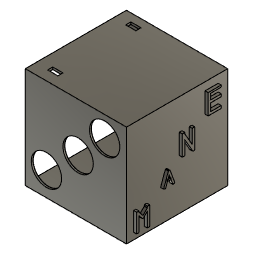
Trabalho #01 (Autodesk Fusion 360 design; units mm, degrees)
Autodesk Fusion 360 part; units mm, degrees
sketch "Sketch1" plane through (0, 0, 0) normal (0, 0, 1) x (1, 0, 0)
  line L0 (2.4742, 2.2756) -> (97.4742, 2.2756)
  line L1 (97.4742, 2.2756) -> (97.4742, 97.2756)
  line L2 (97.4742, 97.2756) -> (2.4742, 97.2756)
  line L3 (2.4742, 97.2756) -> (2.4742, 2.2756)
  line L4 (0, 0) -> (100, 0)
  line L5 (100, 0) -> (100, 100)
  line L6 (100, 100) -> (0, 100)
  line L7 (0, 100) -> (0, 0)
  dimension "d1" = 95
  dimension "d2" = 95
  dimension "d3" = 100
  dimension "d4" = 100
  constraint horizontal L0
  constraint vertical L1
  constraint horizontal L2
  constraint vertical L3
  constraint horizontal L4
  constraint vertical L5
  constraint horizontal L6
  constraint vertical L7
  constraint coincident L4.start L7.end
  measures "d1" distance of L0.start L0.end
  measures "d2" distance of L0.start L2.end
  measures "d3" distance of L4.start L4.end
  measures "d4" distance of L4.start L6.end
extrude "Extrude1" add sketch "Sketch1" along normal blind 113 contours L0 L1 L2 L3 makes body 1
sketch "Sketch2" plane through (0, 0, 0) normal (0, 0, 1) x (1, 0, 0)
  line L0 (0, 0) -> (100, 0)
  line L1 (100, 0) -> (100, 100)
  line L2 (100, 100) -> (0, 100)
  line L3 (0, 100) -> (0, 0)
  dimension "d7" = 100
  dimension "d8" = 100
  constraint horizontal L0
  constraint vertical L1
  constraint horizontal L2
  constraint vertical L3
  constraint coincident L0.start L3.end
  measures "d7" distance of L0.start L0.end
  measures "d8" distance of L0.start L2.end
extrude "Extrude2" cut sketch "Sketch2" along normal blind 113.5 bodies 1
sketch "Sketch3" plane through (0, 0, 0) normal (0, 1, 0) x (1, 0, 0)
  line L0 (0, 0) -> (100, 0)
  line L1 (100, 0) -> (100, -100)
  line L2 (100, -100) -> (0, -100)
  line L3 (0, -100) -> (0, 0)
  dimension "d11" = 100
  dimension "d12" = 100
  constraint horizontal L0
  constraint vertical L1
  constraint horizontal L2
  constraint vertical L3
  constraint coincident L0.start L3.end
  measures "d11" distance of L0.start L0.end
  measures "d12" distance of L0.start L2.end
extrude "Extrude3" add sketch "Sketch3" along normal blind 100 bodies 1
sketch "Sketch4" plane through (0, 0, 0) normal (0, 0, 1) x (1, 0, 0)
  line L0 (0, 0) -> (-96, 0)
  line L1 (-96, 0) -> (-96, -96)
  line L2 (-96, -96) -> (0, -96)
  line L3 (0, -96) -> (0, 0)
  dimension "d15" = 96
  dimension "d16" = 96
  constraint horizontal L0
  constraint vertical L1
  constraint horizontal L2
  constraint vertical L3
  constraint coincident L0.start L3.end
  measures "d15" distance of L0.start L0.end
  measures "d16" distance of L0.start L2.end
extrude "Extrude4" add sketch "Sketch4" along normal blind 96 separate body makes body 2
move_body "Move1" bodies 2 to x (1, 0, 0) y (0, 1, 0) z (0, 0, 1) at (51.5618, 26.4933, 12.8191)
move_body "Move2" bodies 2 to x (1, 0, 0) y (0, 1, 0) z (0, 0, 1) at (30.545, 71.415, -8.7648)
move_body "Move3" bodies 2 to x (1, 0, 0) y (0, 1, 0) z (0, 0, 1) at (-126.1069, -2.5329, 0.0199)
move_body "Move4" bodies 2 to x (1, 0, 0) y (0, 1, 0) z (0, 0, 1) at (14.4031, -1.4043, 59.8669)
move_body "Move5" bodies 2 to x (1, 0, 0) y (0, 1, 0) z (0, 0, 1) at (-24.3693, 162.9476, 0)
move_body "Move6" bodies 2 to x (1, 0, 0) y (0, 1, 0) z (0, 0, 1) at (110, 0, 0)
move_body "Move7" bodies 2 to x (1, 0, 0) y (0, 1, 0) z (0, 0, 1) at (0, -160, -65)
move_body "Move8" bodies 2 to x (1, 0, 0) y (0, 1, 0) z (0, 0, 1) at (0.0912, 0.7995, 1.9212)
move_body "Move9" bodies 2 to x (1, 0, 0) y (0, 1, 0) z (0, 0, 1) at (42.5, 0, 1)
sketch "Sketch5" plane through (0, 0, 0) normal (1, 0, 0) x (0, 1, 0)
  line L0 (97.8521, 97.8156) -> (1.8521, 97.8156)
  line L1 (1.8521, 97.8156) -> (1.8521, 1.8156)
  line L2 (1.8521, 1.8156) -> (97.8521, 1.8156)
  line L3 (97.8521, 1.8156) -> (97.8521, 97.8156)
  dimension "d28" = 96
  dimension "d29" = 96
  constraint horizontal L0
  constraint vertical L1
  constraint horizontal L2
  constraint vertical L3
  measures "d28" distance of L0.start L0.end
  measures "d29" distance of L0.start L2.end
extrude "Extrude5" cut sketch "Sketch5" along normal blind 95 bodies 1 2
hole "Hole1" at (20.9298, 0, 23.8487) direction (0, 1, 0) diameter 30 depth 35 tip angle 118 bodies 1 2
hole "Hole2" at (52.2111, 0, 51.9891) direction (0, 1, 0) diameter 30 depth 35 tip angle 118 bodies 1 2
hole "Hole3" at (78.4554, 0, 79.5683) direction (0, 1, 0) diameter 30 depth 35 tip angle 118 bodies 1 2
sketch "Sketch6" plane through (0, 0, 0) normal (0, 1, 0) x (1, 0, 0)
  line L0 (85.2903, -92.6993, -1.4495) -> (81.4771, -92.6993, -1.4495)
  line L1 (81.4771, -92.6993, -1.4495) -> (81.4771, -68.7847, -1.4495)
  line L2 (81.4771, -68.7847, -1.4495) -> (85.2903, -68.7847, -1.4495)
  line L3 (85.2903, -68.7847, -1.4495) -> (85.2903, -92.6993, -1.4495)
  line L4 (85.2903, -68.7847, -1.4495) -> (68.9975, -68.7847, -1.4495)
  line L5 (68.9975, -68.7847, -1.4495) -> (68.9975, -72.9437, -1.4495)
  line L6 (68.9975, -72.9437, -1.4495) -> (85.2903, -72.9437, -1.4495)
  line L7 (85.2903, -72.9437, -1.4495) -> (85.2903, -68.7847, -1.4495)
extrude "Extrude6" cut sketch "Sketch6" along normal blind 124 contours L0 L1 L3 L6 | L1 L2 L3 L4 L6 L7 | L1 L4 L5 L6 in plane through (0, -1.4495, 0) normal (0, 1, 0) bodies 1
sketch "Sketch7" plane through (0, 0, 0) normal (0, 1, 0) x (1, 0, 0)
  line L0 (60.0969, -63.1547, 3.8658) -> (56.6948, -63.1547, 3.8658)
  line L1 (56.6948, -63.1547, 3.8658) -> (56.6948, -40.1904, 3.8658)
  line L2 (56.6948, -40.1904, 3.8658) -> (60.0969, -40.1904, 3.8658)
  line L3 (60.0969, -40.1904, 3.8658) -> (60.0969, -63.1547, 3.8658)
  line L4 (60.0969, -63.1547, 3.8658) -> (46.0069, -63.1547, 3.8658)
  line L5 (46.0069, -63.1547, 3.8658) -> (46.0069, -60.4679, 3.8658)
  line L6 (46.0069, -60.4679, 3.8658) -> (60.0969, -60.4679, 3.8658)
  line L7 (60.0969, -60.4679, 3.8658) -> (60.0969, -63.1547, 3.8658)
  line L8 (60.0969, -40.1904, 3.8658) -> (46.0069, -40.1904, 3.8658)
  line L9 (46.0069, -40.1904, 3.8658) -> (46.0069, -43.0589, 3.8658)
  line L10 (46.0069, -43.0589, 3.8658) -> (60.0969, -43.0589, 3.8658)
  line L11 (60.0969, -43.0589, 3.8658) -> (60.0969, -40.1904, 3.8658)
  line L12 (60.0969, -54.2007, 3.8658) -> (46.0069, -54.2007, 3.8658)
  line L13 (46.0069, -54.2007, 3.8658) -> (46.0069, -51.6725, 3.8658)
  line L14 (46.0069, -51.6725, 3.8658) -> (60.0969, -51.6725, 3.8658)
  line L15 (60.0969, -51.6725, 3.8658) -> (60.0969, -54.2007, 3.8658)
extrude "Extrude7" cut sketch "Sketch7" along normal blind 130 contours L0 L1 L3 L4 L6 L7 | L1 L4 L5 L6 | L1 L3 L6 L12 | L1 L3 L12 L14 L15 | L1 L12 L13 L14 | L1 L3 L10 L14 | L1 L2 L3 L8 L10 L11 | L1 L8 L9 L10 in plane through (0, 3.8658, 0) normal (0, 1, 0) bodies 1
sketch "Sketch8" plane through (0, 0, 0) normal (0, 1, 0) x (1, 0, 0)
  line L0 (21.525, -36.6076, -1.3332) -> (18.8302, -35.8855, -1.3332)
  line L1 (18.8302, -35.8855, -1.3332) -> (25.0662, -12.6127, -1.3332)
  line L2 (25.0662, -12.6127, -1.3332) -> (27.7609, -13.3347, -1.3332)
  line L3 (27.7609, -13.3347, -1.3332) -> (21.525, -36.6076, -1.3332)
  line L4 (19.0808, -36.5002, -1.3332) -> (12.8449, -13.2273, -1.3332)
  line L5 (21.7756, -35.7781, -1.3332) -> (19.0808, -36.5002, -1.3332)
  line L6 (15.5397, -12.5053, -1.3332) -> (21.7756, -35.7781, -1.3332)
  line L7 (12.8449, -13.2273, -1.3332) -> (15.5397, -12.5053, -1.3332)
  line L8 (22.9646, -20.4557, -1.3332) -> (18.0389, -20.4557, -1.3332)
  line L9 (18.0389, -20.4557, -1.3332) -> (18.0389, -21.8326, -1.3332)
  line L10 (18.0389, -21.8326, -1.3332) -> (22.9646, -21.8326, -1.3332)
  line L11 (22.9646, -21.8326, -1.3332) -> (22.9646, -20.4557, -1.3332)
extrude "Extrude8" cut sketch "Sketch8" along normal blind 105 contours L0 L1 L3 L4 L5 L6 | L1 L2 L3 L6 L10 L11 | L1 L4 L6 L7 | L1 L8 L9 L10 in plane through (0, -1.3332, 0) normal (0, 1, 0) bodies 1
sketch "Sketch9" plane through (0, 0, 0) normal (1, 0, 0) x (0, 1, 0)
sketch "Sketch10" plane through (0, 0, 0) normal (0, 0, 1) x (1, 0, 0)
  line L0 (12.1383, 92.1413, 16.8226) -> (22.1383, 92.1413, 16.8226)
  line L1 (22.1383, 92.1413, 16.8226) -> (22.1383, 87.1413, 16.8226)
  line L2 (22.1383, 87.1413, 16.8226) -> (12.1383, 87.1413, 16.8226)
  line L3 (12.1383, 87.1413, 16.8226) -> (12.1383, 92.1413, 16.8226)
  line L4 (62.606, 94.3283) -> (72.606, 94.3283)
  line L5 (72.606, 94.3283) -> (72.606, 89.3283)
  line L6 (72.606, 89.3283) -> (62.606, 89.3283)
  line L7 (62.606, 89.3283) -> (62.606, 94.3283)
  dimension "d47" = 10
  dimension "d48" = 5
  dimension "d49" = 10
  dimension "d50" = 5
  constraint horizontal L4
  constraint vertical L5
  constraint horizontal L6
  constraint vertical L7
  measures "d49" distance of L4.start L4.end
  measures "d50" distance of L4.start L6.end
extrude "Extrude9" cut sketch "Sketch10" along normal blind 90 contours L0 L1 L2 L3 in plane through (0, 0, 16.8226) normal (0, 0, 1) bodies 1 2
sketch "Sketch11" plane through (0, 0, 100) normal (0, 0, 1) x (-1, 0, 0)
  line L0 (-12.1383, -87.1413) -> (-12.1383, -92.1413)
  line L1 (-12.1383, -92.1413) -> (-22.1383, -92.1413)
  line L2 (-22.1383, -92.1413) -> (-22.1383, -87.1413)
  line L3 (-22.1383, -87.1413) -> (-12.1383, -87.1413)
  line L4 (0, 0) -> (-100, 0)
  line L5 (-100, 0) -> (-100, -100)
  line L6 (-100, -100) -> (0, -100)
  line L7 (0, -100) -> (0, 0)
  line L8 (-12.1383, -10.0064) -> (-22.1383, -10.0064)
  line L9 (-22.1383, -10.0064) -> (-22.1383, -15.0064)
  line L10 (-22.1383, -15.0064) -> (-12.1383, -15.0064)
  line L11 (-12.1383, -15.0064) -> (-12.1383, -10.0064)
  dimension "d53" = 10
  dimension "d54" = 5
  constraint horizontal L8
  constraint vertical L9
  constraint horizontal L10
  constraint vertical L11
  measures "d53" distance of L8.start L8.end
  measures "d54" distance of L8.start L10.end
sketch "Sketch12" plane through (100, 0, 0) normal (1, 0, 0) x (0, 1, 0)
  line L0 (0, 100) -> (0, 0)
  line L1 (0, 0) -> (100, 0)
  line L2 (100, 0) -> (100, 100)
  line L3 (100, 100) -> (0, 100)
  line L4 (7.0299, 25.0937) -> (9.3993, 25.0937)
  line L5 (9.3993, 25.0937) -> (9.3993, 6.5566)
  line L6 (9.3993, 6.5566) -> (7.0299, 6.5566)
  line L7 (7.0299, 6.5566) -> (7.0299, 25.0937)
  line L8 (7.2567, 23.452) -> (8.7515, 24.7063)
  line L9 (8.7515, 24.7063) -> (14.7092, 17.6061)
  line L10 (14.7092, 17.6061) -> (13.2145, 16.3519)
  line L11 (13.2145, 16.3519) -> (7.2567, 23.452)
  line L12 (18.5982, 24.5362) -> (19.978, 23.1565)
  line L13 (19.978, 23.1565) -> (13.4241, 16.6026)
  line L14 (13.4241, 16.6026) -> (12.0444, 17.9823)
  line L15 (12.0444, 17.9823) -> (18.5982, 24.5362)
  line L16 (17.6248, 24.9403) -> (19.9942, 24.9403)
  line L17 (19.9942, 24.9403) -> (19.9942, 6.4031)
  line L18 (19.9942, 6.4031) -> (17.6248, 6.4031)
  line L19 (17.6248, 6.4031) -> (17.6248, 24.9403)
  line L20 (37.9929, 44.4859) -> (39.8368, 45.1571)
  line L21 (39.8368, 45.1571) -> (44.7587, 31.6345)
  line L22 (44.7587, 31.6345) -> (42.9147, 30.9633)
  line L23 (42.9147, 30.9633) -> (37.9929, 44.4859)
  line L24 (38.567, 45.0773) -> (40.411, 44.4062)
  line L25 (40.411, 44.4062) -> (35.4892, 30.8836)
  line L26 (35.4892, 30.8836) -> (33.6452, 31.5548)
  line L27 (33.6452, 31.5548) -> (38.567, 45.0773)
  line L28 (37.1734, 37.6242) -> (41.0282, 37.6242)
  line L29 (41.0282, 37.6242) -> (41.0282, 36.1465)
  line L30 (41.0282, 36.1465) -> (37.1734, 36.1465)
  line L31 (37.1734, 36.1465) -> (37.1734, 37.6242)
  line L32 (52.1474, 69.6446) -> (54.6474, 69.6446)
  line L33 (54.6474, 69.6446) -> (54.6474, 49.6446)
  line L34 (54.6474, 49.6446) -> (52.1474, 49.6446)
  line L35 (52.1474, 49.6446) -> (52.1474, 69.6446)
  line L36 (64.4583, 49.4838) -> (61.9583, 49.4838)
  line L37 (64.4583, 69.4838) -> (64.4583, 49.4838)
  line L38 (61.9583, 49.4838) -> (61.9583, 69.4838)
  line L39 (61.9583, 69.4838) -> (64.4583, 69.4838)
  line L40 (51.9299, 68.0178) -> (54.095, 69.2678)
  line L41 (54.095, 69.2678) -> (65.095, 50.2152)
  line L42 (65.095, 50.2152) -> (62.9299, 48.9652)
  line L43 (62.9299, 48.9652) -> (51.9299, 68.0178)
  line L44 (77.6311, 92.2015) -> (80.1311, 92.2015)
  line L45 (80.1311, 92.2015) -> (80.1311, 72.2015)
  line L46 (80.1311, 72.2015) -> (77.6311, 72.2015)
  line L47 (77.6311, 72.2015) -> (77.6311, 92.2015)
  line L48 (77.6311, 92.2015) -> (90.6311, 92.2015)
  line L49 (90.6311, 92.2015) -> (90.6311, 90.4015)
  line L50 (90.6311, 90.4015) -> (77.6311, 90.4015)
  line L51 (77.6311, 90.4015) -> (77.6311, 92.2015)
  line L52 (77.6311, 72.2015) -> (90.6311, 72.2015)
  line L53 (90.6311, 72.2015) -> (90.6311, 74.7015)
  line L54 (90.6311, 74.7015) -> (77.6311, 74.7015)
  line L55 (77.6311, 74.7015) -> (77.6311, 72.2015)
  line L56 (77.6311, 82.2015) -> (90.6311, 82.2015)
  line L57 (90.6311, 82.2015) -> (90.6311, 84.7015)
  line L58 (90.6311, 84.7015) -> (77.6311, 84.7015)
  line L59 (77.6311, 84.7015) -> (77.6311, 82.2015)
  dimension "d55" = 2.5
  dimension "d56" = 20
  dimension "d57" = 2.5
  dimension "d58" = 20
  dimension "d59" = 2.5
  dimension "d60" = 22
  dimension "d61" = 2.5
  dimension "d62" = 20
  dimension "d63" = 13
  dimension "d64" = 1.8
  dimension "d65" = 13
  dimension "d66" = 2.5
  dimension "d67" = 13
  dimension "d68" = 2.5
  constraint horizontal L4
  constraint vertical L5
  constraint horizontal L6
  constraint vertical L7
  constraint horizontal L16
  constraint vertical L17
  constraint horizontal L18
  constraint vertical L19
  constraint horizontal L28
  constraint vertical L29
  constraint horizontal L30
  constraint vertical L31
  constraint coincident L23 L29.end
  constraint horizontal L32
  constraint vertical L33
  constraint horizontal L34
  constraint vertical L35
  constraint horizontal L39
  constraint vertical L37
  constraint horizontal L36
  constraint vertical L38
  constraint horizontal L44
  constraint vertical L45
  constraint horizontal L46
  constraint vertical L47
  constraint horizontal L48
  constraint vertical L49
  constraint horizontal L50
  constraint vertical L51
  constraint horizontal L52
  constraint vertical L53
  constraint horizontal L54
  constraint vertical L55
  constraint horizontal L56
  constraint vertical L57
  constraint horizontal L58
  constraint vertical L59
  constraint midpoint L47 L56.start
  measures "d55" distance of L32.start L32.end
  measures "d56" distance of L32.start L34.end
  measures "d57" distance of L37.start L38.end
  measures "d58" distance of L36.end L38.end
  measures "d59" distance of L40.start L40.end
  measures "d60" distance of L40.start L42.end
  measures "d61" distance of L44.start L44.end
  measures "d62" distance of L44.start L46.end
  measures "d63" distance of L44.start L48.end
  measures "d64" distance of L44.start L50.end
  measures "d65" distance of L46.end L52.end
  measures "d66" distance of L46.end L54.end
  measures "d67" distance of L56.start L56.end
  measures "d68" distance of L56.start L58.end
extrude "Extrude10" add sketch "Sketch12" along normal blind 3 contours L4 L5 L6 L7 L8 L9 L11 | L5 L9 L10 L11 L13 L14 L15 | L5 L8 L9 L11 | L9 L13 L15 L19 | L9 L13 L14 L15 | L12 L13 L15 L16 L17 L18 L19 | L12 L13 L15 L19 | L20 L21 L23 L24 L25 L27 | L23 L25 L26 L27 L28 L30 L31 | L21 L22 L23 L25 L28 L29 | L23 L25 L28 L30 | L32 L33 L35 L40 L41 | L33 L35 L40 L41 L43 | L33 L38 L41 L43 | L33 L34 L35 L43 | L36 L37 L38 L41 L42 L43 | L37 L38 L39 L41 | L44 L45 L47 L48 L50 L51 | L45 L48 L49 L50 | L45 L47 L50 L58 | L45 L47 L56 L58 L59 | L45 L56 L57 L58 | L45 L47 L54 L56 | L45 L46 L47 L52 L54 L55 | L45 L52 L53 L54 bodies 1 2
extrude "Extrude11" cut sketch "Sketch11" against normal blind 10 contours L8 L9 L10 L11 bodies 1 2
